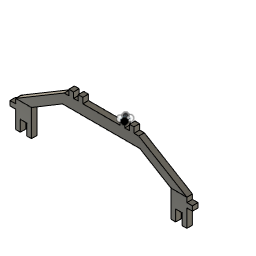
Test Carry Legs v5 (Autodesk Fusion 360 design; units mm, degrees)
Autodesk Fusion 360 part; units mm, degrees
note: some values were not read from the file. Set by a fixed rule: which sketch regions a step uses.
sketch "Sketch1" plane through (0, 0, 0) normal (0, 0, 1) x (1, 0, 0) in component "sidelegs"
  line L0 (-75, -45) -> (-92, -45)
  line L1 (-92, -45) -> (-92, -39)
  line L2 (-92, -39) -> (-75, -39)
  line L3 (-75, -39) -> (-75, -45)
  line L4 (75, -45) -> (92, -45)
  line L5 (92, -45) -> (92, -39)
  line L6 (92, -39) -> (75, -39)
  line L7 (75, -39) -> (75, -45)
  dimension "d7" = 17
  dimension "d8" = 6
  dimension "d9" = 17
  dimension "d10" = 6
  constraint horizontal L0
  constraint vertical L1
  constraint horizontal L2
  constraint vertical L3
  constraint horizontal L4
  constraint vertical L5
  constraint horizontal L6
  constraint vertical L7
  measures "d7" distance of L0.start L0.end
  measures "d8" distance of L0.start L2.end
  measures "d9" distance of L4.start L4.end
  measures "d10" distance of L4.start L6.end
extrude "Extrude1" add sketch "Sketch1" along normal blind 17 makes body 1 at (-80.6667, -45, 11.3333) makes body 2 at (86.3333, -39, 11.3333) in component "sidelegs"
sketch "Sketch2" plane through (0, -45, 0) normal (0, -1, 0) x (1, 0, 0) in component "sidelegs"
  line L0 (-92, 0) -> (-75, 0)
  line L1 (-75, 0) -> (-75, 17)
  line L2 (-75, 17) -> (-92, 17)
  line L3 (-92, 17) -> (-92, 0)
  line L4 (-75, 17) -> (-41.5705, 37.0865)
  line L5 (-75, 17) -> (-36, 17) construction
  line L6 (75, 17) -> (41.5705, 37.0865)
  line L7 (75, 17) -> (114, 17) construction
  line L8 (-41.5705, 37.0865) -> (41.5705, 37.0865)
  line L9 (92, 17) -> (40.2293, 48.107)
  line L10 (40.2293, 48.107) -> (-39.7707, 48.107)
  line L11 (-39.7707, 48.107) -> (-92, 17)
  line L12 (75, 17) -> (92, 17)
  line L13 (-75, 17) -> (-92, 17)
  dimension "d13" = 39
  dimension "d14" = 31
  dimension "d15" = 149
  dimension "d16" = 39
  dimension "d25" = 80
  constraint horizontal L5
  constraint coincident L1.end L2.start
  constraint horizontal L7
  constraint coincident L7 L9.start
  constraint parallel L6 L9
  constraint parallel L7 L10
  constraint coincident L2.end L3.start
  measures "d13" distance of L1.end L4.end
  measures "d14" angle of L4 L5
  measures "d15" angle of L6 L7
  measures "d16" distance of L6.start L6.end
  measures "d25" distance of L9.end L10.end
extrude "Extrude2" add sketch "Sketch2" against normal blind 6 separate body contours L2 L4 L6 L8 L9 L10 L11 L12 L13 makes body 3 in component "sidelegs"
sketch "Sketch3" plane through (0, 0, 0) normal (0, 0, -1) x (1, 0, 0) in component "sidelegs"
  line L0 (-92, 39) -> (-75, 39)
  line L1 (-75, 39) -> (-75, 45)
  line L2 (-75, 45) -> (-92, 45)
  line L3 (-92, 45) -> (-92, 39)
  line L4 (-92, 45) -> (-87, 45)
  line L5 (-87, 45) -> (-87, 39)
  line L6 (-87, 39) -> (-92, 39)
  line L7 (-92, 39) -> (-92, 45)
  line L8 (-75, 45) -> (-80, 45)
  line L9 (-80, 45) -> (-80, 39)
  line L10 (-80, 39) -> (-75, 39)
  line L11 (-75, 39) -> (-75, 45)
  constraint horizontal L4
  constraint vertical L5
  constraint horizontal L6
  constraint vertical L7
  constraint coincident L0 L5.end
  constraint coincident L2.end L3.start
  constraint horizontal L8
  constraint vertical L9
  constraint horizontal L10
  constraint vertical L11
  constraint coincident L0 L9.end
  constraint coincident L1.end L2.start
extrude "Extrude3" add sketch "Sketch3" along normal blind 12 contours L0 L2 L3 L4 L5 L6 L7 | L0 L1 L2 L8 L9 L10 L11 bodies 1 in component "sidelegs"
ref_plane "WorkPlane1" through (0, 0, 0) normal (1, 0, 0) x (0, 1, 0) in component "sidelegs"
sketch "Sketch4" plane through (0, 0, 0) normal (0, 0, -1) x (1, 0, 0) in component "sidelegs"
  line L0 (75, 45) -> (75, 39)
  line L1 (75, 39) -> (92, 39)
  line L2 (92, 39) -> (92, 45)
  line L3 (92, 45) -> (75, 45)
  line L4 (92, 39) -> (87, 39)
  line L5 (87, 39) -> (87, 45)
  line L6 (87, 45) -> (92, 45)
  line L7 (92, 45) -> (92, 39)
  line L8 (75, 39) -> (80, 39)
  line L9 (80, 39) -> (80, 45)
  line L10 (80, 45) -> (75, 45)
  line L11 (75, 45) -> (75, 39)
  constraint horizontal L4
  constraint vertical L5
  constraint horizontal L6
  constraint vertical L7
  constraint coincident L3 L5.end
  constraint coincident L1.end L2.start
  constraint horizontal L8
  constraint vertical L9
  constraint horizontal L10
  constraint vertical L11
  constraint coincident L3 L9.end
  constraint coincident L0.end L1.start
extrude "Extrude4" add sketch "Sketch4" along normal blind 12 contours L0 L1 L3 L8 L9 L10 L11 | L1 L2 L3 L4 L5 L6 L7 bodies 2 in component "sidelegs"
sketch "Sketch5" plane through (0, 0, 48.107) normal (0, 0, 1) x (-1, 0, 0) in component "sidelegs"
  line L0 (39.7707, 45) -> (-40.2293, 45)
  line L1 (-40.2293, 45) -> (-40.2293, 39)
  line L2 (-40.2293, 39) -> (39.7707, 39)
  line L3 (39.7707, 39) -> (39.7707, 45)
  line L4 (-40.2293, 45) -> (-35.2293, 45) construction
  line L5 (-35.2293, 45) -> (-35.2293, 39) construction
  line L6 (-35.2293, 39) -> (-40.2293, 39) construction
  line L7 (-40.2293, 39) -> (-40.2293, 45) construction
  line L8 (39.7707, 45) -> (34.7707, 45) construction
  line L9 (34.7707, 45) -> (34.7707, 39) construction
  line L10 (34.7707, 39) -> (39.7707, 39) construction
  line L11 (39.7707, 39) -> (39.7707, 45) construction
  line L12 (-35.2293, 45) -> (-30.2293, 45) construction
  line L13 (-30.2293, 45) -> (-30.2293, 39) construction
  line L14 (-30.2293, 39) -> (-35.2293, 39) construction
  line L15 (-35.2293, 39) -> (-35.2293, 45) construction
  line L16 (-30, 45) -> (-25, 45) construction
  line L17 (-25, 45) -> (-25, 39) construction
  line L18 (-25, 39) -> (-30, 39) construction
  line L19 (-30, 39) -> (-30, 45) construction
  line L20 (34.7707, 45) -> (29.7707, 45) construction
  line L21 (29.7707, 45) -> (29.7707, 39) construction
  line L22 (29.7707, 39) -> (34.7707, 39) construction
  line L23 (34.7707, 39) -> (34.7707, 45) construction
  line L24 (29.7707, 45) -> (24.7707, 45) construction
  line L25 (24.7707, 45) -> (24.7707, 39) construction
  line L26 (24.7707, 39) -> (29.7707, 39) construction
  line L27 (29.7707, 39) -> (29.7707, 45) construction
  line L28 (34.7707, 45) -> (29.7707, 45)
  line L29 (29.7707, 45) -> (29.7707, 39)
  line L30 (29.7707, 39) -> (34.7707, 39)
  line L31 (34.7707, 39) -> (34.7707, 45)
  line L32 (-35.2293, 45) -> (-30, 45)
  line L33 (-30, 45) -> (-30, 39)
  line L34 (-30, 39) -> (-35.2293, 39)
  line L35 (-35.2293, 39) -> (-35.2293, 45)
  line L36 (-25, 45) -> (-20, 45)
  line L37 (-20, 45) -> (-20, 39)
  line L38 (-20, 39) -> (-25, 39)
  line L39 (-25, 39) -> (-25, 45)
  line L40 (24.7707, 45) -> (19.7707, 45)
  line L41 (19.7707, 45) -> (19.7707, 39)
  line L42 (19.7707, 39) -> (24.7707, 39)
  line L43 (24.7707, 39) -> (24.7707, 45)
  dimension "d26" = 5
  dimension "d27" = 5
  dimension "d28" = 5
  dimension "d29" = 5
  dimension "d30" = 5
  dimension "d31" = 5
  dimension "d32" = 5
  constraint horizontal L4
  constraint vertical L5
  constraint horizontal L6
  constraint vertical L7
  constraint coincident L2 L5.end
  constraint coincident L0.end L1.start
  constraint horizontal L8
  constraint vertical L9
  constraint horizontal L10
  constraint vertical L11
  constraint coincident L2 L9.end
  constraint coincident L0.start L3.end
  constraint horizontal L12
  constraint vertical L13
  constraint horizontal L14
  constraint vertical L15
  constraint coincident L2 L13.end
  constraint horizontal L16
  constraint vertical L17
  constraint horizontal L18
  constraint vertical L19
  constraint coincident L0 L16.start
  constraint horizontal L20
  constraint vertical L21
  constraint horizontal L22
  constraint vertical L23
  constraint coincident L2 L21.end
  constraint horizontal L24
  constraint vertical L25
  constraint horizontal L26
  constraint vertical L27
  constraint coincident L2 L25.end
  constraint horizontal L28
  constraint vertical L29
  constraint horizontal L30
  constraint vertical L31
  constraint horizontal L32
  constraint vertical L33
  constraint horizontal L34
  constraint vertical L35
  constraint horizontal L36
  constraint vertical L37
  constraint horizontal L38
  constraint vertical L39
  constraint coincident L2 L37.end
  constraint horizontal L40
  constraint vertical L41
  constraint horizontal L42
  constraint vertical L43
  measures "d26" distance of L0.end L4.end
  measures "d27" distance of L0.start L8.end
  measures "d28" distance of L4.end L12.end
  measures "d29" distance of L16.start L16.end
  measures "d30" distance of L8.end L20.end
  measures "d31" distance of L20.end L24.end
  measures "d32" distance of L24.end L40.end
extrude "Extrude5" add sketch "Sketch5" along normal blind 6 contours L0 L2 L28 L29 L30 L31 | L0 L2 L40 L41 L42 L43 | L0 L2 L36 L37 L38 L39 | L0 L2 L32 L33 L34 L35 bodies 3 in component "sidelegs"
sketch "Sketch6" plane through (-92, 0, 0) normal (-1, 0, 0) x (0, -1, 0) in component "sidelegs"
  line L0 (45, -12) -> (45, 17)
  line L1 (45, 17) -> (39, 17)
  line L2 (39, 17) -> (39, -12)
  line L3 (39, -12) -> (45, -12)
  line L4 (45, 17) -> (45, 0) construction
  line L5 (39, 0) -> (39, 17) construction
  line L6 (39, 17) -> (45, 17) construction
  line L7 (45, 17) -> (45, 12) construction
  line L8 (45, 12) -> (39, 12) construction
  line L9 (39, 12) -> (39, 17) construction
  line L10 (39, 12) -> (45, 12)
  line L11 (45, 12) -> (45, 7)
  line L12 (45, 7) -> (39, 7)
  line L13 (39, 7) -> (39, 12)
  constraint coincident L0.end L1.start
  constraint coincident L0 L4.end
  constraint perpendicular L1 L4
  constraint coincident L2 L5.start
  constraint coincident L1.end L2.start
  constraint horizontal L6
  constraint vertical L7
  constraint horizontal L8
  constraint vertical L9
  constraint coincident L4 L7.end
  constraint horizontal L10
  constraint vertical L11
  constraint horizontal L12
  constraint vertical L13
  constraint coincident L4 L11.end
extrude "Extrude6" add sketch "Sketch6" along normal blind 6 contours L0 L2 L10 L11 L12 L13 bodies 1 in component "sidelegs"
sketch "Sketch7" plane through (92, 0, 0) normal (1, 0, 0) x (0, 1, 0) in component "sidelegs"
  line L0 (-39, -12) -> (-39, 17)
  line L1 (-39, 17) -> (-45, 17)
  line L2 (-45, 17) -> (-45, -12)
  line L3 (-45, -12) -> (-39, -12)
  line L4 (-45, 17) -> (-39, 17) construction
  line L5 (-39, 17) -> (-39, 12) construction
  line L6 (-39, 12) -> (-45, 12) construction
  line L7 (-45, 12) -> (-45, 17) construction
  line L8 (-45, 12) -> (-39, 12)
  line L9 (-39, 12) -> (-39, 7)
  line L10 (-39, 7) -> (-45, 7)
  line L11 (-45, 7) -> (-45, 12)
  constraint horizontal L4
  constraint vertical L5
  constraint horizontal L6
  constraint vertical L7
  constraint coincident L0 L5.end
  constraint coincident L1.end L2.start
  constraint horizontal L8
  constraint vertical L9
  constraint horizontal L10
  constraint vertical L11
  constraint coincident L0 L9.end
extrude "Extrude7" add sketch "Sketch7" along normal blind 6 contours L0 L2 L8 L9 L10 L11 bodies 2 in component "sidelegs"
sketch "Sketch8" plane through (0, 0, 54.107) normal (0, 0, 1) x (-1, 0, 0) in component "sidelegs"
  line L0 (-35.2293, 39) -> (-30, 39)
  line L1 (-30, 39) -> (-30, 45)
  line L2 (-30, 45) -> (-35.2293, 45)
  line L3 (-35.2293, 45) -> (-35.2293, 39)
  line L4 (-30, 42) -> (-30.229, 42) construction
  line L5 (-30.229, 42) -> (-30.229, 39) construction
  line L6 (-30.229, 42) -> (-30.229, 45) construction
  line L7 (-30.229, 45) -> (-30, 45) construction
  line L8 (-30, 45) -> (-30, 39) construction
  line L9 (-30, 39) -> (-30.229, 39) construction
  line L10 (-30.229, 39) -> (-30.229, 45) construction
  line L11 (-30, 45) -> (-30.229, 45)
  line L12 (-30.229, 45) -> (-30.229, 39)
  line L13 (-30.229, 39) -> (-30, 39)
  line L14 (-30, 39) -> (-30, 45)
  dimension "d39" = 0.229
  constraint midpoint L1 L4.start
  constraint perpendicular L1 L4
  constraint coincident L0 L5.end
  constraint perpendicular L0 L5
  constraint coincident L2 L6.end
  constraint perpendicular L2 L6
  constraint horizontal L7
  constraint vertical L8
  constraint horizontal L9
  constraint vertical L10
  constraint coincident L0.end L1.start
  constraint horizontal L11
  constraint vertical L12
  constraint horizontal L13
  constraint vertical L14
  measures "d39" distance of L4.start L4.end
extrude "Extrude8" cut sketch "Sketch8" against normal blind 6 contours L0 L1 L2 L11 L12 L13 L14 bodies 3 in component "sidelegs"
sketch "Sketch9" plane through (0, 0, 54.107) normal (0, 0, 1) x (-1, 0, 0) in component "sidelegs"
  line L0 (-25, 39) -> (-20, 39)
  line L1 (-20, 39) -> (-20, 45)
  line L2 (-20, 45) -> (-25, 45)
  line L3 (-25, 45) -> (-25, 39)
  line L4 (-25, 45) -> (-25.229, 45)
  line L5 (-25.229, 45) -> (-25.229, 39)
  line L6 (-25.229, 39) -> (-25, 39)
  line L7 (-20.229, 45) -> (-20.229, 39)
  dimension "d42" = 0.229
  dimension "d43" = 6
  dimension "d46" = 0.229
  constraint horizontal L4
  constraint vertical L5
  constraint horizontal L6
  constraint coincident L2.end L3.start
  constraint vertical L7
  constraint coincident L0 L7.end
  measures "d42" distance of L2.end L4.end
  measures "d43" distance of L2.end L0.start
  measures "d46" distance of L1.end L7.start
extrude "Extrude9" add sketch "Sketch9" against normal blind 6 contours L3 L4 L5 L6 bodies 3 in component "sidelegs"
extrude "Extrude10" cut sketch "Sketch9" against normal blind 6 contours L0 L1 L2 L7 bodies 3 in component "sidelegs"
component "sidelegs" placed x (1, 0, 0) y (0, 1, 0) z (0, 0, 1) at (0, 0, 0)
